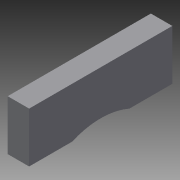
# Autodesk Inventor part: RailMount2x4_NERDS
Saved by Autodesk Inventor 2014 (Build 180170000, 170)
## iProperties
Created: 2016-01-30
Part Number: RailMount2x4_NERDS
Material: Generic
Document SubType Name: Modeling
Designer: bermudezr
Density: 1 g/cm^3
Appearance: Default
Author: bermudezr
Autodesk Inventor part; units mm, degrees
ref_plane "YZ Plane" through (0, 0, 0) normal (1, 0, 0) x (0, 1, 0)
ref_plane "XZ Plane" through (0, 0, 0) normal (0, 1, 0) x (-1, 0, 0)
ref_plane "XY Plane" through (0, 0, 0) normal (0, 0, 1) x (1, 0, 0)
sketch "Sketch1" plane through (0, 0, 0) normal (0, 0, 1) x (1, 0, 0)
  line L0 (-16.6819, 17.4202) -> (21.4181, 17.4202)
  line L1 (21.4181, 17.4202) -> (21.4181, -71.4798)
  line L2 (21.4181, -71.4798) -> (-16.6819, -71.4798)
  line L3 (-16.6819, -71.4798) -> (-16.6819, 17.4202)
  point P0 (0, 0)
  dimension "d0" = 38.1
  dimension "d1" = 88.9
  constraints: 8 end point, 2 parallel, 1 horizontal, 1 perpendicular
  measures "d0" distance of L1.end L2.end
  measures "d1" distance of L0.end L1.end
extrude "Extrusion1" add sketch "Sketch1" along normal blind 254
sketch "Sketch2" plane through (21.4181, -71.4798, 0) normal (1, 0, 0) x (0, 0, -1)
  line L0 (0, 0) -> (-254, 0) projected
  arc A0 (-76.2, 0) -> (-177.8, 0) centre (-127, -116.3974) ccw
  point P0 (0, 71.4798)
  dimension "d4" = 127
  dimension "d5" = 76.2
  dimension "d6" = 76.2
  constraints: 2 point on circle, 2 point on line, 1 centre point
  measures "d4" radius of A0
  measures "d5" distance of L0.end A0.end
  measures "d6" distance of L0.start A0.start
extrude "Extrusion2" cut sketch "Sketch2" against normal blind 76.2
equation "\"d6\" = d5"
body "Solid1"
